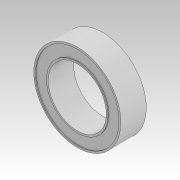
# Autodesk Inventor part: MR128 bearing
Saved by Autodesk Inventor 2020 (Build 240168000, 168)
## iProperties
Created: 2020-11-25
Part Number: MR128 bearing
Material: Generic
Document SubType Name: Modeling
Designer: DDeGo
Density: 1 g/cm^3
Appearance: Default
Author: DDeGo
Autodesk Inventor part; units mm, degrees
ref_plane "YZ Plane" through (0, 0, 0) normal (1, 0, 0) x (0, 1, 0)
ref_plane "XZ Plane" through (0, 0, 0) normal (0, 1, 0) x (-1, 0, 0)
ref_plane "XY Plane" through (0, 0, 0) normal (0, 0, 1) x (1, 0, 0)
sketch "Sketch1" plane through (0, 0, 0) normal (1, 0, 0) x (0, 1, 0)
  line L0 (0, 0) -> (0, -2.1848) construction
  line L1 (0, 0) -> (4, 0) construction
  line L2 (4, 0) -> (4, -1.75)
  line L3 (4, -1.75) -> (4.25, -1.75)
  line L4 (4.25, -1.75) -> (4.25, -1.65)
  line L5 (4.25, -1.65) -> (5.75, -1.65)
  line L6 (5.75, -1.65) -> (5.75, -1.75)
  line L7 (5.75, -1.75) -> (6, -1.75)
  line L8 (6, -1.75) -> (6, 0)
  line L9 (6, 0) -> (4, 0) construction
  line L10 (4, 0) -> (4, 1.75)
  line L11 (4, 1.75) -> (4.25, 1.75)
  line L12 (4.25, 1.75) -> (4.25, 1.65)
  line L13 (4.25, 1.65) -> (5.75, 1.65)
  line L14 (5.75, 1.65) -> (5.75, 1.75)
  line L15 (5.75, 1.75) -> (6, 1.75)
  line L16 (6, 1.75) -> (6, 0)
  dimension "d0" = 4
  dimension "d1" = 6
  dimension "d2" = 0.1
  dimension "d3" = 1.5
  dimension "d6" = 3.5
  constraints: 34 end point, 7 perpendicular, 6 symmetric about line, 5 point on line, 1 collinear, 1 horizontal, 1 vertical
  measures "d0" distance between parallel lines of L0 L2
  measures "d1" distance between parallel lines of L0 L8
  measures "d2" distance between parallel lines of L7 L5
  measures "d3" distance of L4.end L5.end
  measures "d6" distance between parallel lines of L3 L11
revolve "Revolution1" add sketch "Sketch1" angle 360 about axis through (0, 0, 0) along (0, 0, -1)
body "Solid1"
